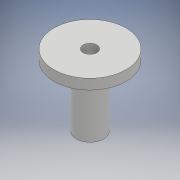
# Autodesk Inventor part: SubSprocketNoTeeth
Saved by Autodesk Inventor 2017 (Build 210142000, 142)
## iProperties
Created: 2016-09-24
Part Number: SubSprocketNoTeeth
Material: Generic
Document SubType Name: Modeling
Designer: vslabsal
Density: 1 g/cm^3
Appearance: Default
Author: vslabsal
Autodesk Inventor part; units mm, degrees
ref_plane "YZ Plane" through (0, 0, 0) normal (1, 0, 0) x (0, 1, 0)
ref_plane "XZ Plane" through (0, 0, 0) normal (0, 1, 0) x (-1, 0, 0)
ref_plane "XY Plane" through (0, 0, 0) normal (0, 0, 1) x (1, 0, 0)
sketch "Sketch1" plane through (0, 0, 0) normal (0, 0, 1) x (1, 0, 0)
  circle A0 centre (0, 0) radius 12.7
  dimension "d0" = 25.4
  constraints: 1 centre point, 1 coincident
  measures "d0" diameter of A0
extrude "Extrusion1" add sketch "Sketch1" along normal blind 56.896
sketch "Sketch2" plane through (0, 0, 56.896) normal (0, 0, 1) x (1, 0, 0)
  circle A0 centre (0, 0) radius 6.35
  dimension "d4" = 12.7
  constraints: 1 centre point, 1 coincident
  measures "d4" diameter of A0
hole "Hole1" at (0, 0, 56.896) direction (0, 0, -1) diameter 12.7 end through all
sketch "Sketch5" plane through (0, 0, 56.896) normal (0, 0, 1) x (1, 0, 0)
  circle A0 centre (0, 0) radius 33.5915
  dimension "d12" = 67.183
  constraints: 1 centre point, 1 coincident
  measures "d12" diameter of A0
extrude "Extrusion2" add sketch "Sketch5" along normal blind 9.525
sketch "Sketch6" plane through (0, 0, 66.421) normal (0, 0, 1) x (1, 0, 0)
  circle A0 centre (0, 0) radius 6.35
  constraints: 1 centre point, 1 coincident
hole "Hole2" at (0, 0, 66.421) direction (0, 0, -1) diameter 12.7 end through all
body "Solid1"
